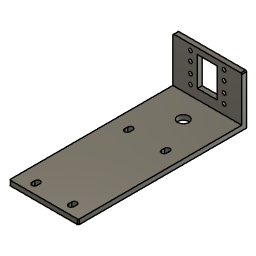
picam3-mount-v2 (Autodesk Fusion 360 design; units mm, degrees)
Autodesk Fusion 360 part; units mm, degrees
sketch "Sketch1" plane through (0, 0, 0) normal (0, 1, 0) x (1, 0, 0)
  line L0 (21.5, 52.5) -> (-21.5, 52.5)
  line L1 (-21.5, 52.5) -> (-21.5, -52.5)
  line L2 (-21.5, -52.5) -> (21.5, -52.5)
  line L3 (21.5, -52.5) -> (21.5, 52.5)
  line L4 (21.5, 52.5) -> (-21.5, -52.5) construction
  line L5 (-21.5, 52.5) -> (21.5, -52.5) construction
  dimension "d1" = 43
  dimension "d2" = 105
  constraint horizontal L0
  constraint perpendicular L0 L1
  constraint parallel L0 L2
  constraint parallel L1 L3
  constraint coincident L4 origin
  constraint coincident L5 origin
  measures "d1" distance of L1.end L2.end
  measures "d2" distance of L0.end L1.end
extrude "Extrude1" add sketch "Sketch1" along normal blind 3
sketch "Sketch2" plane through (0, 3, 0) normal (0, 1, 0) x (-1, 0, 0)
  line L0 (-21.5, 52.5) -> (-21.5, -52.5)
  line L1 (-21.5, -52.5) -> (21.5, -52.5)
  line L2 (21.5, -52.5) -> (21.5, 52.5)
  line L3 (21.5, 52.5) -> (-21.5, 52.5)
  line L4 (15, -14.5) -> (-15, -14.5) construction
  line L5 (-15, -14.5) -> (-15, 50.5) construction
  line L6 (-15, 50.5) -> (15, 50.5) construction
  line L7 (15, 50.5) -> (15, -14.5) construction
  line L8 (-13.1, 47) -> (-13.1, 45)
  arc A0 (-13.1, 45) -> (-9.9, 45) centre (-11.5, 45) ccw
  line L9 (-9.9, 45) -> (-9.9, 47)
  arc A1 (-9.9, 47) -> (-13.1, 47) centre (-11.5, 47) ccw
  line L10 (-11.5, 47) -> (-11.5, 45) construction
  line L11 (0, 20) -> (0, 2.5)
  arc A2 (13.1, 47) -> (9.9, 47) centre (11.5, 47) ccw
  line L12 (13.1, 47) -> (13.1, 45)
  line L13 (9.9, 45) -> (9.9, 47)
  arc A3 (9.9, 45) -> (13.1, 45) centre (11.5, 45) ccw
  line L14 (-15, 18) -> (15, 18) construction
  arc A4 (-9.9, -11) -> (-13.1, -11) centre (-11.5, -11) ccw
  line L15 (-13.1, -11) -> (-13.1, -13)
  line L16 (-9.9, -13) -> (-9.9, -11)
  arc A5 (-13.1, -13) -> (-9.9, -13) centre (-11.5, -13) ccw
  line L17 (0, 1.75) -> (0, 22.5)
  line L18 (9.9, -13) -> (9.9, -11)
  arc A6 (13.1, -11) -> (9.9, -11) centre (11.5, -11) ccw
  line L19 (13.1, -11) -> (13.1, -13)
  arc A7 (9.9, -13) -> (13.1, -13) centre (11.5, -13) ccw
  dimension "d10" = 30
  dimension "d11" = 65
  dimension "d12" = 2
  dimension "d13" = 6.5
  dimension "d15" = 2
  dimension "d16" = 3.2
  dimension "d17" = 3.5
  dimension "d18" = 3.5
  dimension "d19" = 2
  dimension "d20" = 3.2
  dimension "d21" = 56
  constraint horizontal L4
  constraint perpendicular L4 L5
  constraint parallel L4 L6
  constraint parallel L5 L7
  constraint tangent L8 A0
  constraint tangent A0 L9
  constraint parallel L8 L9
  constraint tangent L9 A1
  constraint tangent L8 A1
  constraint parallel L5 L10
  constraint symmetric L8.start L11 A2.start
  constraint symmetric L8.end L11 L12.end
  constraint symmetric A0.end L11 L13.start
  constraint symmetric L9.end L11 A2.end
  constraint symmetric A0 L11 A3
  constraint symmetric A1 L11 A2
  constraint coincident L5 L14.start
  constraint coincident L7 L14.end
  constraint perpendicular L7 L14
  constraint midpoint L5 L14.start
  constraint tangent L15 A5
  constraint tangent L16 A5
  constraint parallel L15 L16
  constraint tangent A4 L16
  constraint tangent A4 L15
  constraint symmetric A4.end L17 A6.start
  constraint symmetric L16.start L17 L18.start
  constraint symmetric L15.end L17 L19.end
  constraint symmetric A4.start L17 L18.end
  constraint symmetric A4 L17 A6
  constraint symmetric A5 L17 A7
  measures "d10" distance of L5.end L6.end
  measures "d11" distance of L4.start L6.end
  measures "d12" distance of L3 L6
  measures "d13" distance of L0 L5
  measures "d15" distance of A1.centre A0.centre
  measures "d16" diameter of A0
  measures "d17" distance of L5 A1.centre
  measures "d18" distance of L6 A1.centre
  measures "d19" distance of A5.centre A4.centre
  measures "d20" diameter of A5
  measures "d21" distance of A0.centre A4.centre
extrude "Extrude2" cut sketch "Sketch2" against normal blind 4 contours L8 A0 L9 A1 | A2 L12 L13 A3 | A4 L15 L16 A5 | L18 A6 L19 A7
sketch "Sketch3" plane through (0, 3, 0) normal (0, 1, 0) x (-1, 0, 0)
  line L0 (-9.9, -11) -> (-9.9, -13)
  arc A0 (-13.1, -13) -> (-9.9, -13) centre (-11.5, -13) ccw
  line L1 (-13.1, -13) -> (-13.1, -11)
  arc A1 (-9.9, -11) -> (-13.1, -11) centre (-11.5, -11) ccw
  line L2 (-13.1, 45) -> (-13.1, 47)
  arc A2 (-9.9, 47) -> (-13.1, 47) centre (-11.5, 47) ccw
  line L3 (-9.9, 47) -> (-9.9, 45)
  arc A3 (-13.1, 45) -> (-9.9, 45) centre (-11.5, 45) ccw
  line L4 (9.9, 45) -> (9.9, 47)
  arc A4 (13.1, 47) -> (9.9, 47) centre (11.5, 47) ccw
  line L5 (13.1, 47) -> (13.1, 45)
  arc A5 (9.9, 45) -> (13.1, 45) centre (11.5, 45) ccw
  line L6 (-21.5, 52.5) -> (-21.5, -52.5)
  line L7 (-21.5, -52.5) -> (21.5, -52.5)
  line L8 (21.5, -52.5) -> (21.5, 52.5)
  line L9 (21.5, 52.5) -> (-21.5, 52.5)
  line L10 (-21.5, -52.5) -> (21.5, -52.5)
  line L11 (21.5, -52.5) -> (21.5, -49.5)
  line L12 (21.5, -49.5) -> (-21.5, -49.5)
  line L13 (-21.5, -49.5) -> (-21.5, -52.5)
  line L14 (9.9, -13) -> (9.9, -11)
  arc A6 (13.1, -11) -> (9.9, -11) centre (11.5, -11) ccw
  line L15 (13.1, -11) -> (13.1, -13)
  arc A7 (9.9, -13) -> (13.1, -13) centre (11.5, -13) ccw
  dimension "d24" = 3
  constraint horizontal L10
  constraint vertical L11
  constraint horizontal L12
  constraint vertical L13
  constraint coincident L8 L11.end
  constraint coincident L6.end L7.start
  measures "d24" distance of L6.end L12.end
extrude "Extrude3" add sketch "Sketch3" along normal blind 28 contours L6 L7 L8 L10 L11 L12 L13
sketch "Sketch4" plane through (0, 0, -49.5) normal (0, 0, 1) x (1, 0, 0)
  line L0 (-21.5, 3) -> (21.5, 3)
  line L1 (21.5, 3) -> (21.5, 31)
  line L2 (21.5, 31) -> (-21.5, 31)
  line L3 (-21.5, 31) -> (-21.5, 3)
  line L4 (6.2, 27.4) -> (-6.2, 27.4)
  line L5 (-6.2, 27.4) -> (-6.2, 9)
  line L6 (-6.2, 9) -> (6.2, 9)
  line L7 (6.2, 9) -> (6.2, 27.4)
  line L8 (0, 2.5) -> (0, 20)
  line L9 (-10.5, 27.4) -> (10.5, 27.4) construction
  circle A0 centre (-10.5, 27.4) radius 1.15
  circle A1 centre (10.5, 27.4) radius 1.15
  line L10 (-10.5, 14.9) -> (10.5, 14.9) construction
  circle A2 centre (-10.5, 14.9) radius 1.15
  circle A3 centre (10.5, 14.9) radius 1.15
  line L11 (-6.2, 18.2) -> (6.2, 18.2)
  circle A4 centre (10.5, 9) radius 1.15
  circle A5 centre (-10.5, 21.5) radius 1.15
  circle A6 centre (-10.5, 9) radius 1.15
  circle A7 centre (10.5, 21.5) radius 1.15
  line L12 (6.2, 27.4) -> (6.2, 9)
  line L13 (-6.2, 27.4) -> (6.2, 27.4)
  line L14 (-6.2, 9) -> (-6.2, 27.4)
  line L15 (6.2, 9) -> (-6.2, 9)
  dimension "d27" = 12.4
  dimension "d28" = 6.2
  dimension "d29" = 18.4
  dimension "d30" = 6
  dimension "d33" = 2.3
  dimension "d34" = 2.3
  dimension "d35" = 12.5
  dimension "d38" = 2.3
  dimension "d39" = 2.3
  dimension "d40" = 21
  dimension "d41" = 21
  dimension "d42" = 10.5
  constraint horizontal L4
  constraint vertical L5
  constraint horizontal L6
  constraint vertical L7
  constraint parallel L2 L9
  constraint coincident L4.end L9
  constraint coincident L9.start A0.centre
  constraint coincident L9.end A1.centre
  constraint horizontal L10
  constraint coincident L10.start A2.centre
  constraint coincident L10.end A3.centre
  constraint midpoint L5 L11.start
  constraint midpoint L7 L11.end
  constraint symmetric L4.start L11 L6.end
  constraint symmetric L4.end L11 L5.end
  constraint symmetric L5.end L11 L4.end
  constraint symmetric L6.end L11 L4.start
  constraint symmetric A0 L11 A6
  constraint symmetric A1 L11 A4
  constraint symmetric A2 L11 A5
  constraint symmetric A3 L11 A7
  measures "d27" distance of L5.end L6.end
  measures "d28" distance of L5 L8
  measures "d29" distance of L4 L6
  measures "d30" distance of L0 L6
  measures "d33" diameter of A0
  measures "d34" diameter of A1
  measures "d35" distance of L9 L10
  measures "d38" diameter of A2
  measures "d39" diameter of A3
  measures "d40" distance of L9.start L9.end
  measures "d41" distance of L10.start L10.end
  measures "d42" horizontal distance of L8.end L9.end
extrude "Extrude4" cut sketch "Sketch4" against normal up to surface (3 mm away) contours L4 L5 L7 L11 L12 L13 L14 | L6 L7 L8 L11 L12 L15 | L5 L6 L8 L11 L14 L15 | A0 | A1 | A2 | A3 | A4 | A5 | A6 | A7
sketch "Sketch5" plane through (0, 3, 0) normal (0, 1, 0) x (-1, 0, 0)
  line L0 (-21.5, 52.5) -> (-21.5, -49.5)
  line L1 (-21.5, -49.5) -> (21.5, -49.5)
  line L2 (21.5, -49.5) -> (21.5, 52.5)
  line L3 (-9.9, -11) -> (-9.9, -13)
  arc A0 (-13.1, -13) -> (-9.9, -13) centre (-11.5, -13) ccw
  line L4 (-13.1, -13) -> (-13.1, -11)
  arc A1 (-9.9, -11) -> (-13.1, -11) centre (-11.5, -11) ccw
  line L5 (-13.1, 45) -> (-13.1, 47)
  arc A2 (-9.9, 47) -> (-13.1, 47) centre (-11.5, 47) ccw
  line L6 (-9.9, 47) -> (-9.9, 45)
  arc A3 (-13.1, 45) -> (-9.9, 45) centre (-11.5, 45) ccw
  line L7 (9.9, 45) -> (9.9, 47)
  arc A4 (13.1, 47) -> (9.9, 47) centre (11.5, 47) ccw
  line L8 (13.1, 47) -> (13.1, 45)
  arc A5 (9.9, 45) -> (13.1, 45) centre (11.5, 45) ccw
  circle A6 centre (0, -34.5) radius 3.5
  line L9 (9.9, -13) -> (9.9, -11)
  arc A7 (13.1, -11) -> (9.9, -11) centre (11.5, -11) ccw
  line L10 (13.1, -11) -> (13.1, -13)
  arc A8 (9.9, -13) -> (13.1, -13) centre (11.5, -13) ccw
  line L11 (21.5, 52.5) -> (-21.5, 52.5)
  dimension "d49" = 7
  dimension "d55" = 15
  measures "d49" diameter of A6
  measures "d55" vertical distance of L1.end A6.centre
extrude "Extrude6" cut sketch "Sketch5" against normal up to surface (3 mm away) contours A6
fillet "Fillet3" radius 0.6 4 edges at (21.5, 1.5, 52.5) (-21.5, 1.5, 52.5) (-21.5, 31, -51) (21.5, 31, -51)
